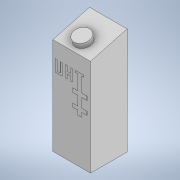
# Autodesk Inventor part: milch
Saved by Autodesk Inventor 2021 (Build 250183000, 183)
## iProperties
Created: 2021-07-22
Part Number: milch
Material: Generisch
Document SubType Name: Modeling
Designer: Simon
Density: 1 g/cm^3
Appearance: Vorgabe
Author: Simon
Autodesk Inventor part; units mm, degrees
ref_plane "YZ Plane" through (0, 0, 0) normal (1, 0, 0) x (0, 1, 0)
ref_plane "XZ Plane" through (0, 0, 0) normal (0, 1, 0) x (-1, 0, 0)
ref_plane "XY Plane" through (0, 0, 0) normal (0, 0, 1) x (1, 0, 0)
sketch "Skizze1" plane through (0, 0, 0) normal (0, 0, 1) x (1, 0, 0)
  line L0 (-36.5, 103.5) -> (36.5, 103.5)
  line L1 (36.5, 103.5) -> (36.5, -103.5)
  line L2 (36.5, -103.5) -> (-36.5, -103.5)
  line L3 (-36.5, -103.5) -> (-36.5, 103.5)
  point P0 (0, 0)
  point P1 (0, 103.5)
  point P2 (-36.5, 0)
  dimension "d0" = 73
  dimension "d1" = 207
  constraints: 8 end point, 2 midpoint, 2 parallel, 1 horizontal, 1 horizontal alignment, 1 perpendicular, 1 vertical alignment
  measures "d0" distance between parallel lines of L1 L3
  measures "d1" distance between parallel lines of L2 L0
extrude "Extrusion1" add sketch "Skizze1" along normal mid plane 71
sketch "Skizze2" plane through (0, 0, 35.5) normal (0, 0, 1) x (1, 0, 0)
  line L0 (-31.9691, 54.6598) -> (-31.9691, 32.0411)
  line L1 (-31.9691, 32.0411) -> (-18.3639, 32.0411)
  line L2 (-18.3639, 32.0411) -> (-18.3639, 54.6598)
  line L3 (-18.3639, 54.6598) -> (-22.1053, 54.6598)
  line L4 (-22.1053, 54.6598) -> (-22.1053, 35.4424)
  line L5 (-22.1053, 35.4424) -> (-28.2277, 35.4424)
  line L6 (-28.2277, 35.4424) -> (-28.2277, 54.6598)
  line L7 (-28.2277, 54.6598) -> (-31.9691, 54.6598)
  line L8 (-12.2415, 54.6598) -> (-12.2415, 32.0411)
  line L9 (-12.2415, 32.0411) -> (-8.8402, 32.0411)
  line L10 (-8.8402, 32.0411) -> (-8.8402, 40.7145)
  line L11 (-8.8402, 40.7145) -> (-1.8675, 40.7145)
  line L12 (-1.8675, 40.7145) -> (-1.8675, 32.0411)
  line L13 (-1.8675, 32.0411) -> (1.7039, 32.0411)
  line L14 (1.7039, 32.0411) -> (1.7039, 54.6598)
  line L15 (1.7039, 54.6598) -> (-1.8675, 54.6598)
  line L16 (-1.8675, 45.0511) -> (-1.8675, 54.6598)
  line L17 (-1.8675, 45.0511) -> (-8.8402, 45.0511)
  line L18 (-8.8402, 45.0511) -> (-8.8402, 54.6598)
  line L19 (-12.2415, 54.6598) -> (-8.8402, 54.6598)
  line L20 (7.316, 54.6598) -> (7.316, 51.0885)
  line L21 (7.316, 51.0885) -> (12.0779, 51.0885)
  line L22 (12.0779, 51.0885) -> (12.0779, -18.2168)
  line L23 (12.0779, -18.2168) -> (19.2206, -18.2168)
  line L24 (19.2206, -18.2168) -> (19.2206, 51.0885)
  line L25 (19.2206, 51.0885) -> (23.6423, 51.0885)
  line L26 (23.6423, 51.0885) -> (23.6423, 54.6598)
  line L27 (23.6423, 54.6598) -> (7.316, 54.6598)
  line L28 (1.7039, 22.5174) -> (1.7039, 15.0346)
  line L29 (1.7039, 15.0346) -> (29.5946, 15.0346)
  line L30 (29.5946, 15.0346) -> (29.5946, 22.5174)
  line L31 (29.5946, 22.5174) -> (1.7039, 22.5174)
  line L32 (1.7039, -3.1128) -> (29.5946, -3.1128)
  line L33 (29.5946, -3.1128) -> (29.5946, -9.8501)
  line L34 (29.5946, -9.8501) -> (1.7039, -9.8501)
  line L35 (1.7039, -9.8501) -> (1.7039, -3.1128)
  point P0 (0, 0)
  point P1 (12.0779, 22.5174)
  point P2 (12.0779, 15.0346)
  point P3 (19.2206, 15.0346)
  point P4 (19.2206, 22.5174)
  point P5 (19.2206, -3.1128)
  point P6 (19.2206, -9.8501)
  point P7 (12.0779, -9.8501)
  point P8 (12.0779, -3.1128)
  constraints: 72 end point, 25 perpendicular, 17 point on line, 3 vertical, 2 parallel, 1 horizontal
extrude "Extrusion2" cut sketch "Skizze2" against normal blind 0.1
chamfer "Fase1" distance 71 angle 15 1 edges at (0, 103.5, 35.5) measured on face at (12.1667, 103.5, -11.8333)
sketch "Skizze3" plane through (-36.5, 84.4756, 35.5) normal (0, 0.9659, 0.2588) x (1, 0, 0)
  circle A0 centre (36.5, 22.9067) radius 15.376
  point P0 (36.5, 12.4265)
  constraints: 1 centre point
extrude "Extrusion3" add sketch "Skizze3" along normal blind 10
